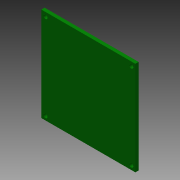
# Autodesk Inventor part: Empty Inner PCB
Saved by Autodesk Inventor 2015 SP1 (Build 190203100, 203)
## iProperties
Created: 2015-06-22
Part Number: Empty Inner PCB
Material: Generic
Document SubType Name: Modeling
Designer: Kartikye
Density: 1 g/cm^3
Appearance: Default
Author: Kartikye
Autodesk Inventor part; units mm, degrees
ref_plane "YZ Plane" through (0, 0, 0) normal (1, 0, 0) x (0, 1, 0)
ref_plane "XZ Plane" through (0, 0, 0) normal (0, 1, 0) x (-1, 0, 0)
ref_plane "XY Plane" through (0, 0, 0) normal (0, 0, 1) x (1, 0, 0)
sketch "Sketch1" plane through (0, 0, 0) normal (0, 1, 0) x (-1, 0, 0)
  line L0 (-23, 23) -> (23, 23)
  line L1 (23, 23) -> (23, -23)
  line L2 (23, -23) -> (-23, -23)
  line L3 (-23, -23) -> (-23, 23)
  line L4 (-23, 23) -> (23, -23) construction
  line L5 (23, 23) -> (-23, -23) construction
  point P0 (0, 0)
  dimension "d0" = 46
  dimension "d1" = 46
  constraints: 12 end point, 2 midpoint, 2 parallel, 1 horizontal, 1 perpendicular
  measures "d0" distance of L1.end L2.end
  measures "d1" distance of L0.end L1.end
extrude "Extrusion1" add sketch "Sketch1" along normal blind 1.6
sketch "Sketch2" plane through (0, 1.6, 0) normal (0, 1, 0) x (1, 0, 0)
  circle A0 centre (21, -21) radius 1
  line L0 (23, -23) -> (23, 23) projected
  line L1 (-23, -23) -> (23, -23) projected
  circle A1 centre (21, 21) radius 1
  circle A2 centre (-21, -21) radius 1
  circle A3 centre (-21, 21) radius 1
  line L2 (23, 23) -> (-23, 23) projected
  line L3 (-23, 23) -> (-23, -23) projected
  point P0 (0, 0)
  dimension "d4" = 2
  dimension "d5" = 2
  dimension "d6" = 2
  dimension "d7" = 2
  dimension "d8" = 2
  dimension "d9" = 2
  dimension "d10" = 2
  dimension "d11" = 2
  dimension "d12" = 2
  dimension "d13" = 2
  dimension "d14" = 2
  dimension "d15" = 2
  constraints: 4 centre point
  measures "d4" diameter of A0
  measures "d5" distance from line of L0 A0.centre
  measures "d6" distance from line of L1 A0.centre
  measures "d7" diameter of A1
  measures "d8" diameter of A2
  measures "d9" diameter of A3
  measures "d10" distance from line of L0 A1.centre
  measures "d11" distance from line of L2 A1.centre
  measures "d12" distance from line of L2 A3.centre
  measures "d13" distance from line of L3 A3.centre
  measures "d14" distance from line of L3 A2.centre
  measures "d15" distance from line of L1 A2.centre
extrude "Extrusion2" cut sketch "Sketch2" against normal blind 1.6 contours A0 | A1 | A2 | A3
body "Solid1"
